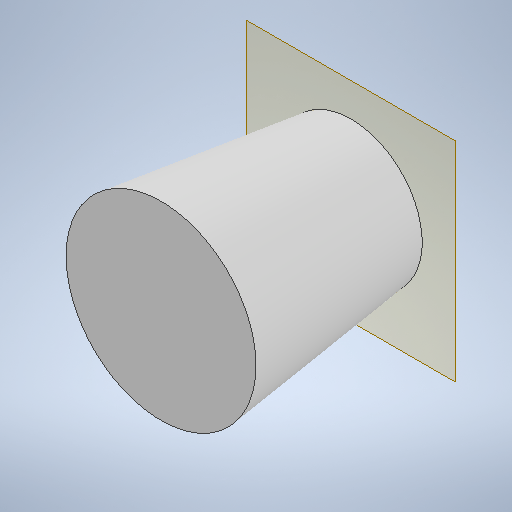
# Autodesk Inventor part: peca_005_001
Saved by Autodesk Inventor 2025.2 (Build 292293000, 293)
## iProperties
Created: 2025-03-25
Part Number: peca_005_001
Material: Genérico
Document SubType Name: Modeling
Designer: Carlos Dias
Density: 1 g/cm^3
Appearance: Padrão
Author: Carlos Dias
Autodesk Inventor part; units mm, degrees
ref_plane "YZ Plane" through (0, 0, 0) normal (1, 0, 0) x (0, 1, 0)
ref_plane "XZ Plane" through (0, 0, 0) normal (0, 1, 0) x (-1, 0, 0)
sketch "Esboço1" plane through (0, 0, 0) normal (0, 0, 1) x (1, 0, 0)
  circle A0 centre (0, 0) radius 50
  dimension "d0" = 100
  constraints: 1 centre point, 1 coincident
  measures "d0" diameter of A0
ref_plane "Plano de trabalho1" through (0, 0, -100) normal (0, 0, 1) x (1, 0, 0)
sketch "Esboço2" plane through (0, 0, -100) normal (0, 0, 1) x (1, 0, 0)
  circle A0 centre (0, 0) radius 37.5
  dimension "d2" = 75
  constraints: 1 centre point, 1 coincident
  measures "d2" diameter of A0
loft "Transição1" add profiles "Esboço2", "Esboço1"
